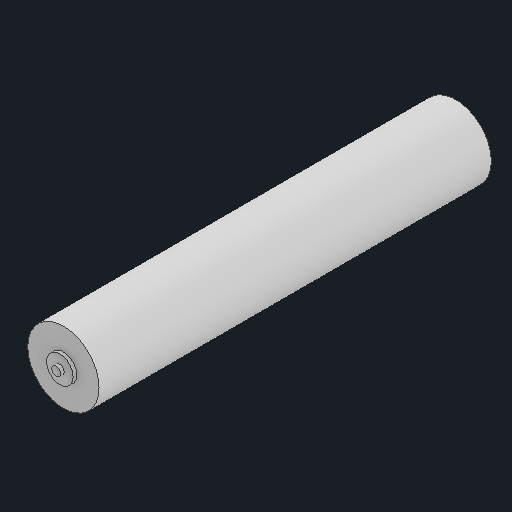
# Autodesk Inventor part: Teste Limpador
Saved by Autodesk Inventor 2026.2 (Build 302298010, 298A)
## iProperties
Created: 2026-02-22
Part Number: Teste Limpador
Material: Generic
Document SubType Name: Modeling
Designer: Rubens
Density: 1 g/cm^3
Appearance: Default
Author: Rubens
Autodesk Inventor part; units mm, degrees
ref_plane "YZ Plane" through (0, 0, 0) normal (1, 0, 0) x (0, 1, 0)
ref_plane "XZ Plane" through (0, 0, 0) normal (0, 1, 0) x (-1, 0, 0)
ref_plane "XY Plane" through (0, 0, 0) normal (0, 0, 1) x (1, 0, 0)
sketch "Sketch1" plane through (0, 0, 0) normal (0, 0, 1) x (1, 0, 0)
  circle A0 centre (0, 0) radius 37.5
  circle A1 centre (0, 0) radius 12.5
  circle A2 centre (0, 0) radius 100
  dimension "d0" = 75
  dimension "d1" = 25
  dimension "d2" = 200
  constraints: 3 centre point, 3 coincident
  measures "d0" diameter of A0
  measures "d1" diameter of A1
  measures "d2" diameter of A2
extrude "Extrusion1" add sketch "Sketch1" against normal blind 1100 contours A2
extrude "Extrusion2" add sketch "Sketch1" along normal blind 10 contours A0
extrude "Extrusion3" add sketch "Sketch1" along normal blind 20 contours A1
body "Solid1"
